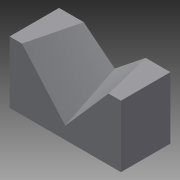
# Autodesk Inventor part: 7.1 Part 3
Saved by Autodesk Inventor 2015 (Build 190159000, 159)
## iProperties
Created: 2015-03-05
Part Number: 7.1 Part 3
Material: Generic
Document SubType Name: Modeling
Designer: PLTW-Stu-02
Density: 1 g/cm^3
Appearance: Default
Author: PLTW-Stu-02
Autodesk Inventor part; units mm, degrees
ref_plane "YZ Plane" through (0, 0, 0) normal (1, 0, 0) x (0, 1, 0)
ref_plane "XZ Plane" through (0, 0, 0) normal (0, 1, 0) x (-1, 0, 0)
ref_plane "XY Plane" through (0, 0, 0) normal (0, 0, 1) x (1, 0, 0)
sketch "Sketch1" plane through (0, 0, 0) normal (0, 0, 1) x (1, 0, 0)
  line L0 (21.3373, 22.3876) -> (111.3373, 22.3876)
  line L1 (111.3373, 22.3876) -> (111.3373, 72.3876)
  line L2 (111.3373, 72.3876) -> (21.3373, 72.3876)
  line L3 (21.3373, 72.3876) -> (21.3373, 22.3876)
  point P0 (0, 0)
  constraints: 8 end point, 2 parallel, 1 horizontal, 1 perpendicular
extrude "Extrusion1" add sketch "Sketch1" along normal blind 40
sketch "Sketch4" plane through (0, 0, 40) normal (0, 0, 1) x (1, 0, 0)
  line L0 (111.3373, 72.3876) -> (21.3373, 72.3876) projected
  line L1 (31.3373, 72.3876) -> (66.3412, 32.3876)
  line L2 (66.3412, 32.3876) -> (101.3373, 72.3876)
  line L3 (21.3373, 72.3876) -> (21.3373, 22.3876) projected
  line L4 (111.3373, 22.3876) -> (111.3373, 72.3876) projected
  line L5 (21.3373, 22.3876) -> (111.3373, 22.3876) projected
  point P0 (0, 0)
  dimension "d14" = 10
  dimension "d15" = 10
  dimension "d16" = 10
  dimension "d17" = 44.9961
  constraints: 4 end point, 2 point on line
  measures "d14" distance from line of L3 L1.start
  measures "d15" distance from line of L4 L2.end
  measures "d16" distance from line of L5 L1.end
  measures "d17" distance from line of L4 L1.end
sketch "Sketch5" plane through (0, 0, 0) normal (0, 0, -1) x (-1, 0, 0)
  line L0 (-111.3373, 72.3876) -> (-21.3373, 72.3876) projected
  line L1 (-91.3373, 72.3876) -> (-66.3334, 52.3876)
  line L2 (-66.3334, 52.3876) -> (-41.3373, 72.3876)
  line L3 (-21.3373, 72.3876) -> (-21.3373, 22.3876) projected
  line L4 (-111.3373, 22.3876) -> (-111.3373, 72.3876) projected
  line L5 (-21.3373, 22.3876) -> (-111.3373, 22.3876) projected
  point P0 (0, 0)
  dimension "d18" = 20
  dimension "d19" = 20
  dimension "d20" = 30
  dimension "d21" = 44.9961
  constraints: 4 end point, 2 point on line
  measures "d18" distance from line of L3 L2.end
  measures "d19" distance from line of L4 L1.start
  measures "d20" distance from line of L5 L1.end
  measures "d21" distance from line of L3 L1.end
loft "Loft1" cut profiles "Sketch4", "Sketch5" contours L2 L1 L0 / L0 L2 L1
body "Solid1"
